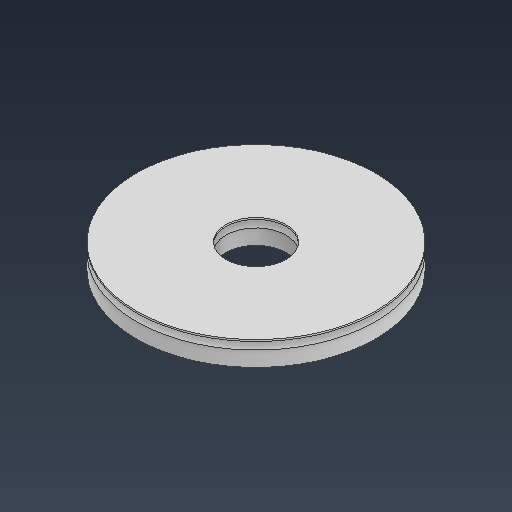
# Autodesk Inventor part: ECB_demo
Saved by Autodesk Inventor 2025.3 (Build 293356000, 356)
## iProperties
Created: 2025-12-02
Part Number: ECB_demo
Material: 一般
Document SubType Name: Modeling
Designer: 陳泓任
Density: 1 g/cm^3
Appearance: 預設
Author: 陳泓任
Autodesk Inventor part; units mm, degrees
ref_plane "YZ Plane" through (0, 0, 0) normal (1, 0, 0) x (0, 1, 0)
ref_plane "XZ Plane" through (0, 0, 0) normal (0, 1, 0) x (-1, 0, 0)
ref_plane "XY Plane" through (0, 0, 0) normal (0, 0, 1) x (1, 0, 0)
sketch "草圖1" plane through (0, 0, 0) normal (0, 1, 0) x (-1, 0, 0)
  circle A0 centre (0, 0) radius 79.3187
  circle A1 centre (0, 0) radius 20
  dimension "d_yo" = 158.6374
  dimension "d_yi" = 40
  constraints: 2 centre point, 2 coincident
  measures "d_yo" diameter of A0
  measures "d_yi" diameter of A1
extrude "擠出1" add sketch "草圖1" along normal blind 10
sketch "草圖2" plane through (0, 10, 0) normal (0, 1, 0) x (1, 0, 0)
  arc A0 (-73.4779, 27.1074) -> (-73.4779, -27.1074) centre (0, 0) ccw
  line L0 (-90.8067, 0) -> (132.5495, 0) construction
  arc A1 (-29.1269, 10.7455) -> (-29.1269, -10.7455) centre (0, 0) ccw
  line L1 (-73.4779, -27.1074) -> (-29.1269, -10.7455)
  line L2 (-29.1269, 10.7455) -> (-73.4779, 27.1074)
  arc A2 (-51.3024, 18.9265) -> (-51.3024, -18.9265) centre (0, 0) ccw construction
  line L3 (-32.7889, -71.1246) -> (-12.9976, -28.194)
  arc A3 (-28.194, -12.9976) -> (-12.9976, -28.194) centre (0, 0) ccw
  line L4 (-28.194, -12.9976) -> (-71.1246, -32.7889)
  arc A4 (-71.1246, -32.7889) -> (-32.7889, -71.1246) centre (0, 0) ccw
  line L5 (27.1074, -73.4779) -> (10.7455, -29.1269)
  arc A5 (-10.7455, -29.1269) -> (10.7455, -29.1269) centre (0, 0) ccw
  line L6 (-10.7455, -29.1269) -> (-27.1074, -73.4779)
  arc A6 (-27.1074, -73.4779) -> (27.1074, -73.4779) centre (0, 0) ccw
  line L7 (71.1246, -32.7889) -> (28.194, -12.9976)
  arc A7 (12.9976, -28.194) -> (28.194, -12.9976) centre (0, 0) ccw
  line L8 (12.9976, -28.194) -> (32.7889, -71.1246)
  arc A8 (32.7889, -71.1246) -> (71.1246, -32.7889) centre (0, 0) ccw
  circle A9 centre (0, 0) radius 20 construction
  line L9 (73.4779, 27.1074) -> (29.1269, 10.7455)
  arc A10 (29.1269, -10.7455) -> (29.1269, 10.7455) centre (0, 0) ccw
  line L10 (29.1269, -10.7455) -> (73.4779, -27.1074)
  arc A11 (73.4779, -27.1074) -> (73.4779, 27.1074) centre (0, 0) ccw
  line L11 (32.7889, 71.1246) -> (12.9976, 28.194)
  arc A12 (28.194, 12.9976) -> (12.9976, 28.194) centre (0, 0) ccw
  line L12 (28.194, 12.9976) -> (71.1246, 32.7889)
  arc A13 (71.1246, 32.7889) -> (32.7889, 71.1246) centre (0, 0) ccw
  line L13 (-27.1074, 73.4779) -> (-10.7455, 29.1269)
  arc A14 (10.7455, 29.1269) -> (-10.7455, 29.1269) centre (0, 0) ccw
  line L14 (10.7455, 29.1269) -> (27.1074, 73.4779)
  arc A15 (27.1074, 73.4779) -> (-27.1074, 73.4779) centre (0, 0) ccw
  line L15 (-71.1246, 32.7889) -> (-28.194, 12.9976)
  arc A16 (-12.9976, 28.194) -> (-28.194, 12.9976) centre (0, 0) ccw
  line L16 (-12.9976, 28.194) -> (-32.7889, 71.1246)
  arc A17 (-32.7889, 71.1246) -> (-71.1246, 32.7889) centre (0, 0) ccw
  point P0 (-22.8933, -49.6593)
  point P1 (-49.6593, -22.8933)
  point P2 (18.9265, -51.3024)
  point P3 (-18.9265, -51.3024)
  point P4 (49.6593, -22.8933)
  point P5 (22.8933, -49.6593)
  point P6 (51.3024, 18.9265)
  point P7 (51.3024, -18.9265)
  point P8 (22.8933, 49.6593)
  point P9 (49.6593, 22.8933)
  point P10 (-18.9265, 51.3024)
  point P11 (18.9265, 51.3024)
  point P12 (-49.6593, 22.8933)
  point P13 (-22.8933, 49.6593)
  dimension "r_av" = 54.6822
  dimension "l_m" = 47.2729
  dimension "d8" = 360
  dimension "theta_magnet" = 40.5
  constraints: 34 end point, 34 point on circle, 17 centre point, 3 line through centre, 2 coincident, 2 midpoint, 1 concentric, 1 horizontal, 1 point on line, 90 other
  measures "r_av" radius of A2
  measures "l_m" distance of L2.start L2.end
  measures "theta_magnet" angle of L2 L1
extrude "擠出3" add sketch "草圖2" along normal blind 2.1078 separate body contours L2 A1 L1 A0
sketch "草圖3" plane through (0, 0, 0) normal (0, 0, 1) x (1, 0, 0)
  line L0 (20, 16.0229) -> (79.3187, 16.0229)
  line L1 (79.3187, 16.0229) -> (79.3187, 14.9344)
  line L2 (79.3187, 14.9344) -> (20, 14.9344)
  line L3 (20, 14.9344) -> (20, 16.0229)
  line L4 (0, 63.9711) -> (0, -11.167) construction
  line L5 (79.3187, 10) -> (-79.3187, 10) projected
  point P0 (0, 0)
  dimension "r_co" = 79.3187
  dimension "r_ci" = 20
  dimension "t_c" = 1.0885
  dimension "gap_low" = 4.9344
  constraints: 10 end point, 2 parallel, 1 horizontal, 1 perpendicular, 1 point on line, 1 vertical
  measures "r_co" distance between parallel lines of L4 L1
  measures "r_ci" distance between parallel lines of L4 L3
  measures "t_c" distance of L0.end L1.end
  measures "gap_low" distance between parallel lines of L5 L2
revolve "迴轉1" add sketch "草圖3" angle 360 about axis through (0, 63.9711, 0) along (0, -1, 0) separate body
equation "\"d_yo\" = 2 * r_yo"
equation "\"d_yi\" = 2 * r_yi"
equation "\"r_co\" = r_yo"
equation "\"r_ci\" = r_yi"
equation "\"r_yo\" = 79.31871"
equation "\"r_yi\" = 20"
equation "\"gap_high\" = 1"
equation "\"theta_p\" = 45deg"
equation "\"PM_ratio\" = 0.9"
